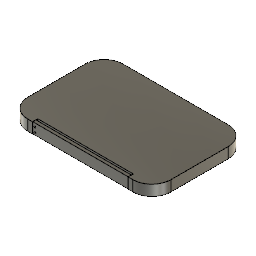
Orthogon v1 v3 (Autodesk Fusion 360 design; units mm, degrees)
Autodesk Fusion 360 part; units mm, degrees
sketch "Sketch1" plane through (0, 0, 0) normal (0, 1, 0) x (1, 0, 0)
  line L0 (40.125, -5.85) -> (34.875, -5.85)
sketch "Sketch2" plane through (0, 0, 0) normal (0, -1, 0) x (1, 0, 0)
  line L0 (5, 5) -> (0, 5)
  line L1 (0, 5) -> (0, 0)
  line L2 (0, 0) -> (5, 0)
  line L3 (5, 0) -> (5, 5)
sketch "Sketch3" plane through (0, 0, 0) normal (0, 0, 1) x (1, 0, 0)
  line L0 (0, 0) -> (75, 0)
  line L1 (75, 0) -> (75, 50)
  line L2 (75, 50) -> (0, 50)
  line L3 (0, 50) -> (0, 0)
  dimension "d5" = 75
  dimension "d6" = 50
  measures "d5" distance of L0.start L0.end
  measures "d6" distance of L0.start L2.end
ref_plane "WorkPlane1" through (0, 0, 0) normal (0, 0, 1) x (1, 0, 0)
sketch "Sketch5" plane through (0, 0, 5.85) normal (0, 0, 1) x (-1, 0, 0)
  arc A0 (-65, 0) -> (-75, -10) centre (-65, -10) ccw
  line L0 (-75, -10) -> (-75, -40)
  arc A1 (-75, -40) -> (-65, -50) centre (-65, -40) ccw
  line L1 (-65, -50) -> (-10, -50)
  arc A2 (-10, -50) -> (0, -40) centre (-10, -40) ccw
  line L2 (0, -40) -> (0, -10)
  arc A3 (0, -10) -> (-10, 0) centre (-10, -10) ccw
  line L3 (-10, 0) -> (-34.875, 0)
  line L4 (-40.125, 0) -> (-65, 0)
  line L5 (-34.875, 0) -> (-40.125, 0)
  line L6 (-12.5, 0.0039) -> (-62.5, 0.0039)
  line L7 (-62.5, 0.0039) -> (-62.5, -2.7261)
  line L8 (-62.5, -2.7261) -> (-12.5, -2.7261)
  line L9 (-12.5, -2.7261) -> (-12.5, 0.0039)
  line L10 (-12.5, 0.0039) -> (-62.5, -2.7261) construction
  line L11 (-62.5, 0.0039) -> (-12.5, -2.7261) construction
  point P0 (-51.415, 0)
  point P1 (-18.335, 0)
  point P2 (-37.5, -1.3611)
  dimension "d58" = 50
  dimension "d59" = 2.73
  measures "d58" distance of L7.end L8.end
  measures "d59" distance of L6.end L7.end
extrude "Extrude11" add sketch "Sketch5" along normal blind 5.64 contours A0 L0 A1 L1 A2 L2 A3 L3 L4 L7 L8 L9 makes body 1
ref_plane "WorkPlane2" through (0, 0, 5.85) normal (0, 0, 1) x (1, 0, 0)
sketch "Sketch7" plane through (0, 0, 0) normal (0, 1, 0) x (1, 0, 0)
  line L0 (0, 0) -> (50, 0)
  line L1 (50, 0) -> (50, -5.6)
  line L2 (50, -5.6) -> (0, -5.6)
  line L3 (0, -5.6) -> (0, 0)
  line L4 (9.2, 0) -> (12.7, 0)
  line L5 (12.7, 0) -> (12.7, -3.5)
  line L6 (12.7, -3.5) -> (9.2, -3.5)
  line L7 (9.2, -3.5) -> (9.2, 0)
  line L8 (23.7, 0) -> (23.7, -3.5)
  line L9 (23.7, -3.5) -> (20.2, -3.5)
  line L10 (20.2, -3.5) -> (20.2, 0)
  line L11 (20.2, 0) -> (23.7, 0)
  line L12 (34.7, 0) -> (34.7, -3.5)
  line L13 (34.7, -3.5) -> (31.2, -3.5)
  line L14 (31.2, -3.5) -> (31.2, 0)
  line L15 (31.2, 0) -> (34.7, 0)
  line L16 (45.7, 0) -> (45.7, -3.5)
  line L17 (45.7, -3.5) -> (42.2, -3.5)
  line L18 (42.2, -3.5) -> (42.2, 0)
  line L19 (42.2, 0) -> (45.7, 0)
  circle A0 centre (1.1, -3.8) radius 0.45
  circle A1 centre (1.1, -1.26) radius 0.45
  dimension "d62" = 50
  dimension "d63" = 5.6
  dimension "d64" = 3.5
  dimension "d65" = 3.5
  dimension "d68" = 11
  dimension "d69" = 0
  dimension "d70" = 0.9
  dimension "d73" = 0
  dimension "d74" = 2.54
  measures "d62" distance of L0.start L0.end
  measures "d63" distance of L0.start L2.end
  measures "d64" distance of L4.start L4.end
  measures "d65" distance of L4.start L6.end
  measures "d70" diameter of A0
extrude "Extrude12" add sketch "Sketch7" along normal blind 1.65 separate body contours L0 L1 L2 L3 L5 L6 L7 L8 L9 L10 L12 L13 L14 L16 L17 L18 makes body 2
extrude "Extrude13" add sketch "Sketch7" along normal blind 1.65 separate body contours L0 L1 L2 L3 L5 L6 L7 L8 L9 L10 L12 L13 L14 L16 L17 L18 | L0 L4 L5 L6 L7 | L0 L8 L9 L10 L11 | L0 L16 L17 L18 L19 | L0 L12 L13 L14 L15 | A0 | A1 makes body 3
extrude "Extrude14" add sketch "Sketch7" along normal blind 1 from surface at 1.65 contours L0 L4 L5 L6 L7 | L0 L8 L9 L10 L11 | L0 L16 L17 L18 L19 | L0 L12 L13 L14 L15 bodies 3 2
extrude "Extrude15" cut sketch "Sketch7" along normal blind 1.65 contours A0 | A1 bodies 3
move_body "Move2" bodies 3 to x (1, 0, 0) y (0, 1, 0) z (0, 0, 1) at (12.54, 0.1, 5.89)
named bodies: "Acrylic body", "LED board"
